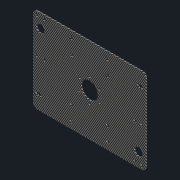
# Autodesk Inventor part: carbon_plate14
Saved by Autodesk Inventor 2021 (Build 250183000, 183)
## iProperties
Created: 2021-08-06
Part Number: carbon_plate14
Material: CFRP
Document SubType Name: Sheet Metal
Designer: yuta0
Density: 1.43 g/cm^3
Sheet Metal Rule: Default_mm
Appearance: カーボンファイバー
Mass: 50.9816 g
Surface Area: 370.557 cm^2
Volume: 35.6515 cm^3
Author: yuta0
Autodesk Inventor part; units mm, degrees
ref_plane "YZ Plane" through (0, 0, 0) normal (1, 0, 0) x (0, 1, 0)
ref_plane "XZ Plane" through (0, 0, 0) normal (0, 1, 0) x (-1, 0, 0)
ref_plane "XY Plane" through (0, 0, 0) normal (0, 0, 1) x (1, 0, 0)
sketch "スケッチ1" plane through (0, 0, 0) normal (0, 0, 1) x (1, 0, 0)
  line L0 (-78, -59) -> (78, -59)
  line L1 (78, -59) -> (78, 59)
  line L2 (78, 59) -> (-78, 59)
  line L3 (-78, 59) -> (-78, -59)
  line L4 (-78, -59) -> (78, 59) construction
  line L5 (78, -59) -> (-78, 59) construction
  point P0 (0, 0)
  dimension "d0" = 156
  dimension "d1" = 118
  measures "d0" distance of L1.end L2.end
  measures "d1" distance of L2.end L0.start
extrude "プレート1" add sketch "スケッチ1" along normal blind 2
sketch "スケッチ2" plane through (0, 0, 2) normal (0, 0, 1) x (1, 0, 0)
  line L0 (-25, 30) -> (25, 30)
  line L1 (25, 30) -> (25, 50)
  line L2 (25, 50) -> (-25, 50)
  line L3 (-25, 50) -> (-25, 30)
  line L4 (-25, 30) -> (25, 50) construction
  line L5 (25, 30) -> (-25, 50) construction
  line L6 (-78, 59) -> (78, 59) projected
  point P0 (0, 0)
  point P1 (0, 40)
  point P2 (0, 40)
  point P3 (0, 40)
  dimension "d3" = 50
  dimension "d4" = 20
  dimension "d60" = 40
  constraints: 12 end point, 4 midpoint, 2 parallel, 1 horizontal, 1 perpendicular, 1 vertical alignment
  measures "d3" distance of L1.end L2.end
  measures "d4" distance of L2.end L0.start
  measures "d60" distance of point (0, 0) point (0, 40)
hole "穴1" at (-25, 50, 2) at (-25, 30, 2) at (25, 30, 2) at (25, 50, 2) direction (0, 0, -1) diameter 4.3 depth 2 clearance for "Flat Head Machine Screw" size "M4" standard "Ansi Metric M Profile"
sketch "スケッチ3" plane through (0, 0, 2) normal (0, 0, 1) x (1, 0, 0)
  line L0 (-63, 5.4) -> (-73, 5.4)
  line L1 (-73, 5.4) -> (-73, 54)
  line L2 (-73, 54) -> (-63, 54)
  line L3 (-63, 54) -> (-63, 5.4)
  line L4 (-63, 5.4) -> (-73, 54) construction
  line L5 (-73, 5.4) -> (-63, 54) construction
  line L6 (-78, 59) -> (78, 59) projected
  line L7 (-78, -59) -> (-78, 59) projected
  circle A0 centre (-68, 40) radius 6
  point P0 (0, 0)
  point P1 (-68, 29.7)
  point P2 (-68, 29.7)
  dimension "d18" = 10
  dimension "d19" = 48.6
  dimension "d20" = 14
  dimension "d31" = 19
  dimension "d47" = 68
  dimension "d48" = 12
  constraints: 12 end point, 3 midpoint, 2 parallel, 1 centre point, 1 coincident, 1 horizontal, 1 perpendicular, 1 vertical alignment
  measures "d18" distance of L1.end L2.end
  measures "d19" distance of L0.end L1.end
  measures "d20" distance from line of L2 point (-68, 40)
  measures "d31" distance from line of L6 point (-68, 40)
  measures "d47" horizontal distance of point (0, 0) point (-68, 40)
  measures "d48" diameter of A0
extrude "押し出し2" cut sketch "スケッチ3" against normal blind 10 contours A0 L1 L3 | L3 A0 | A0 L1
hole "穴2" at (-63, 5.4, 2) at (-73, 5.4, 2) at (-73, 54, 2) at (-63, 54, 2) direction (0, 0, -1) diameter 4.3 depth 2 clearance for "Flat Head Machine Screw" size "M4" standard "Ansi Metric M Profile"
sketch "スケッチ4" plane through (0, 0, 2) normal (0, 0, 1) x (1, 0, 0)
  circle A0 centre (0, 0) radius 16
  point P0 (0, 16)
  point P1 (-13.8564, 8)
  point P2 (-13.8564, -8)
  point P3 (0, -16)
  point P4 (13.8564, -8)
  point P5 (13.8564, 8)
  dimension "d32" = 32
  dimension "d35" = 360
  constraints: 1 coincident, 1 vertical alignment, 9 other
hole "穴3" at (0, 16, 2) at (-13.8564, 8, 2) at (-13.8564, -8, 2) at (0, -16, 2) at (13.8564, -8, 2) at (13.8564, 8, 2) direction (0, 0, -1) diameter 3.2 end through all clearance for "Socket Head Cap Screw" size "M3" standard "Ansi Metric M Profile"
sketch "スケッチ5" plane through (0, 0, 2) normal (0, 0, 1) x (1, 0, 0)
  circle A0 centre (0, 0) radius 12
  dimension "d44" = 24
  constraints: 1 centre point, 1 coincident
  measures "d44" diameter of A0
extrude "押し出し1" cut sketch "スケッチ5" against normal blind 10
sketch "スケッチ6" plane through (0, 0, 2) normal (0, 0, 1) x (1, 0, 0)
  point P0 (0, 0)
sketch "スケッチ7" plane through (0, 0, 2) normal (0, 0, 1) x (1, 0, 0)
  line L0 (68, 40) -> (73, 40) construction
  line L1 (68, 37.85) -> (73, 37.85)
  line L2 (73, 42.15) -> (68, 42.15)
  arc A0 (68, 42.15) -> (68, 37.85) centre (68, 40) ccw
  arc A1 (73, 37.85) -> (73, 42.15) centre (73, 40) ccw
  circle A2 centre (-68, 40) radius 6 projected
  point P0 (0, 0)
  point P1 (70.5, 40)
  dimension "d54" = 2.15
  dimension "d55" = 5
  dimension "d57" = 68
  constraints: 8 end point, 4 point on circle, 4 tangent, 2 centre point, 2 horizontal alignment, 1 midpoint, 1 parallel
  measures "d54" radius of A1
  measures "d55" distance of L0.start L0.end
  measures "d57" horizontal distance of point (0, 0) L0.start
extrude "押し出し3" cut sketch "スケッチ7" against normal blind 10 contours A0 L2 A1 L1
sketch "スケッチ8" plane through (0, 0, 0) normal (0, 0, -1) x (-1, 0, 0)
  point P0 (0, 0)
fillet "コーナーR1" radius 5 4 edges at (-78, 59, 1) (78, 59, 1) (78, -59, 1) (-78, -59, 1)
pattern_circular "円形状パターン1" count 2 over 360 about axis through (0, 0, -10) along (0, 0, 1) of "穴1", "押し出し2", "穴2", "押し出し3"
equation "\"d14\" = Thickness"
equation "\"d28\" = Thickness"
equation "\"d42\" = Thickness"
equation "\"d2\" = Thickness"
equation "\"BendRadius\" = Thickness"
equation "\"BendReliefWidth\" = Thickness"
equation "\"BendReliefDepth\" = 0.5 * Thickness"
equation "\"CornerReliefSize\" = 4 * Thickness"
equation "\"MinimumRemnant\" = 2 * Thickness"
equation "\"TransitionRadius\" = BendRadius"
equation "\"JacobiRadiusSize\" = BendRadius"
equation "\"GapSize\" = Thickness"
equation "\"Thickness\" = 2"
